percolator_cap (Autodesk Fusion 360 design; units mm, degrees)
Autodesk Fusion 360 part; units mm, degrees
note: some values were not read from the file. Set by a fixed rule: which sketch regions a step uses.
sketch "Sketch1" plane through (0, 0, 0) normal (1, 0, 0) x (0, 1, 0)
  line L0 (-8.75, 0) -> (-8.75, 6.9)
  line L1 (0, 0) -> (0, 67)
  line L2 (0, 0) -> (-8.75, 0)
  line L3 (-8.75, 6.9) -> (-12.35, 6.9)
  line L4 (-12.35, 6.9) -> (-12.35, 8.9)
  line L5 (-12.35, 8.9) -> (-8, 23.5)
  line L6 (-5.75, 0) -> (-5.75, 31.5)
  line L7 (-5.75, 31.5) -> (0, 31.5)
  line L8 (0, 0) -> (-13.7425, 0)
  line L9 (-8, 23.5) -> (-8, 31.5)
  line L10 (-8, 31.5) -> (-7.1919, 33.5)
  line L11 (-7.1919, 33.5) -> (0, 33.5)
  dimension "d1" = 8.75
  dimension "d2" = 13.7425
  dimension "d3" = 6.9
  dimension "d4" = 3.6
  dimension "d5" = 2
  dimension "d6" = 3
  dimension "d8" = 31.5
  dimension "d10" = 8
  dimension "d11" = 8
  dimension "d13" = 8
  dimension "d25" = 22
  dimension "d26" = 2
  dimension "d27" = 2
  constraint coincident L1.start L2.start
  constraint vertical L1
  constraint perpendicular L0 L2
  constraint perpendicular L0 L3
  constraint perpendicular L2 L4
  constraint coincident L2 L6.start
  constraint perpendicular L2 L6
  constraint coincident L1 L7.end
  constraint perpendicular L1 L7
  constraint perpendicular L1 L8
  constraint collinear L2 L8
  constraint midpoint L1 L11.end
  measures "d1" horizontal distance of L1.start L0.start
  measures "d2" distance of L1.start L8.end
  measures "d3" distance of L0.start L0.end
  measures "d4" distance of L0.end L3.end
  measures "d5" distance of L3.end L4.end
  measures "d6" distance of L0 L6
  measures "d8" distance of L6.start L6.end
  measures "d10" distance of L1 L9.end
  measures "d11" distance of L1 L5.end
  measures "d13" vertical distance of L5.end L9.end
  measures "d25" angle of L9 L10
  measures "d26" distance of L9.end L11
  measures "d27" distance of L7 L11
revolve "Revolve1" add sketch "Sketch1" angle 360 about axis through (0, 0, 0) along (0, 0, 1) contours L0 L1 L2 L3 L4 L5 L6 L7 L8 L9 L10 L11
sketch "Sketch2" plane through (0, 0, 0) normal (1, 0, 0) x (0, 1, 0)
  line L0 (-8.75, 3) -> (-10.25, 3)
  line L1 (-10.25, 3) -> (-10.25, 0)
  line L2 (-10.25, 0) -> (-8.75, 0)
  line L3 (-8.75, 0) -> (-8.75, 3)
  line L4 (-8.75, 0) -> (-8.75, 6.9)
  line L5 (-8.75, 3) -> (-7.5, 3)
  line L6 (-7.5, 3) -> (-7.5, 0)
  line L7 (-7.5, 0) -> (-8.75, 0)
  line L8 (-8.75, 0) -> (-8.75, 3)
  dimension "d15" = 3
  dimension "d16" = 1.5
  constraint horizontal L0
  constraint vertical L1
  constraint horizontal L2
  constraint vertical L3
  constraint coincident L2.end L4
  constraint coincident L2.end L3.start
  constraint horizontal L5
  constraint vertical L6
  constraint horizontal L7
  constraint vertical L8
  measures "d15" distance of L0.end L1.end
  measures "d16" distance of L0.start L0.end
extrude "Extrude1" add sketch "Sketch2" along normal mid plane 3.5
mirror "Mirror1" about plane through (0, 0, 0) normal (0, 1, 0) of "Revolve1", "Extrude1"
fillet "Fillet1" radius 0.5 6 edges at (-1.75, -10.25, 1.5) (0, -10.25, 3) (1.75, -10.25, 1.5) (1.75, 10.25, 1.5) (0, 10.25, 3) (-1.75, 10.25, 1.5)
chamfer "Chamfer1" distance 1 angle 30 1 edges at (-5.3609, -2.0793, 31.5) measured on face at (-0.5725, -5.7214, 21)
equation "d1 = ( 17.5 / 2 ) * 1 mm"
equation "d17 = ( 3.5 / 2 ) * 1 mm"
